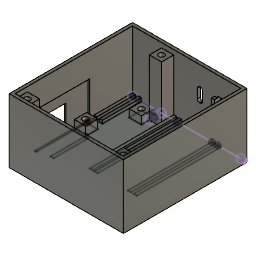
Final_Enclosure (Autodesk Fusion 360 design; units mm, degrees)
Autodesk Fusion 360 part; units mm, degrees
sketch "Sketch1" plane through (0, 0, 0) normal (0, 0, 1) x (1, 0, 0)
  line L0 (0, 0) -> (75, 0)
  line L1 (75, 0) -> (75, 81)
  line L2 (75, 81) -> (0, 81)
  line L3 (0, 81) -> (0, 0)
  dimension "d1" = 81
  dimension "d2" = 75
  constraint horizontal L0
  constraint vertical L1
  constraint horizontal L2
  constraint vertical L3
  constraint coincident L0.start L3.end
  measures "d1" distance of L0.start L2.end
  measures "d2" distance of L0.start L0.end
extrude "Extrude1" add sketch "Sketch1" along normal blind 2 makes body 1
sketch "Sketch2" plane through (0, 0, 2) normal (0, 0, 1) x (-1, 0, 0)
  line L0 (0, -81) -> (0, 0)
  line L1 (0, 0) -> (-75, 0)
  line L2 (-75, 0) -> (-75, -81)
  line L3 (-75, -81) -> (0, -81)
  line L4 (0, 0) -> (-75, 0)
  line L5 (-75, 0) -> (-75, -81)
  line L6 (-75, -81) -> (0, -81)
  line L7 (0, -81) -> (0, 0)
  line L8 (-73, -2) -> (-73, -79)
  line L9 (-73, -79) -> (-2, -79)
  line L10 (-2, -79) -> (-2, -2)
  line L11 (-2, -2) -> (-73, -2)
  dimension "d5" = -2
  constraint horizontal L4
  constraint vertical L5
  constraint horizontal L6
  constraint vertical L7
  constraint coincident L2.end L3.start
  constraint coincident L0.end L1.start
extrude "Extrude2" add sketch "Sketch2" along normal blind 40 bodies 1
sketch "Sketch3" plane through (0, 0, 2) normal (0, 0, 1) x (-1, 0, 0)
  line L0 (-73, -2) -> (-73, -79)
  line L1 (-73, -79) -> (-2, -79)
  line L2 (-2, -79) -> (-2, -2)
  line L3 (-2, -2) -> (-73, -2)
  line L4 (-54, -79) -> (-56, -79)
  line L5 (-56, -79) -> (-56, -24)
  line L6 (-56, -24) -> (-54, -24)
  line L7 (-54, -24) -> (-54, -79)
  line L8 (-57.75, -79) -> (-59.75, -79)
  line L9 (-59.75, -79) -> (-59.75, -24)
  line L10 (-59.75, -24) -> (-57.75, -24)
  line L11 (-57.75, -24) -> (-57.75, -79)
  line L12 (-31, -79) -> (-29, -79)
  line L13 (-29, -79) -> (-29, -24)
  line L14 (-29, -24) -> (-31, -24)
  line L15 (-31, -24) -> (-31, -79)
  line L16 (-34.25, -79) -> (-32.25, -79)
  line L17 (-32.25, -79) -> (-32.25, -24)
  line L18 (-32.25, -24) -> (-34.25, -24)
  line L19 (-34.25, -24) -> (-34.25, -79)
  line L20 (-2, -79) -> (-4, -79)
  line L21 (-4, -79) -> (-4, -53.5)
  line L22 (-4, -53.5) -> (-2, -53.5)
  line L23 (-2, -53.5) -> (-2, -79)
  line L24 (-5.68, -79) -> (-7.68, -79)
  line L25 (-7.68, -79) -> (-7.68, -53.5)
  line L26 (-7.68, -53.5) -> (-5.68, -53.5)
  line L27 (-5.68, -53.5) -> (-5.68, -79)
  line L28 (-9.3, -40.8) -> (-11.3, -40.8)
  line L29 (-11.3, -40.8) -> (-11.3, -18)
  line L30 (-11.3, -18) -> (-9.3, -18)
  line L31 (-9.3, -18) -> (-9.3, -40.8)
  line L32 (-9.3, -40.8) -> (-2, -40.8)
  line L33 (-2, -40.8) -> (-2, -48.8)
  line L34 (-2, -48.8) -> (-9.3, -48.8)
  line L35 (-9.3, -48.8) -> (-9.3, -40.8)
  line L36 (-1, -50.8) -> (-1, -16)
  line L37 (-1, -16) -> (-2, -16)
  line L38 (-2, -16) -> (-2, -48.8)
  line L39 (-1, -50.8) -> (-2, -50.8)
  line L40 (-2, -50.8) -> (-2, -48.8)
  dimension "d8" = 17
  dimension "d9" = 15.25
  dimension "d10" = 2
  dimension "d11" = 2
  dimension "d12" = 55
  dimension "d13" = 25
  dimension "d14" = 23.75
  dimension "d15" = 2
  dimension "d16" = 2
  dimension "d17" = 2
  dimension "d18" = 1.68
  dimension "d19" = 2
  dimension "d20" = 25.5
  dimension "d44" = 7.3
  dimension "d45" = 2
  dimension "d46" = 22.8
  dimension "d47" = 16
  dimension "d48" = 8
  dimension "d49" = 1
  dimension "d50" = 34.8
  dimension "d69" = 2
  constraint horizontal L4
  constraint vertical L5
  constraint horizontal L6
  constraint vertical L7
  constraint coincident L1 L4.start
  constraint horizontal L8
  constraint vertical L9
  constraint horizontal L10
  constraint vertical L11
  constraint coincident L1 L8.start
  constraint horizontal L5.end L10.end
  constraint horizontal L12
  constraint vertical L13
  constraint horizontal L14
  constraint vertical L15
  constraint coincident L1 L12.start
  constraint horizontal L16
  constraint vertical L17
  constraint horizontal L18
  constraint vertical L19
  constraint horizontal L14.end L18.end
  constraint horizontal L6.end L18.end
  constraint horizontal L20
  constraint vertical L21
  constraint horizontal L22
  constraint vertical L23
  constraint coincident L1.end L2.start
  constraint horizontal L24
  constraint vertical L25
  constraint horizontal L26
  constraint vertical L27
  constraint coincident L1 L24.start
  constraint horizontal L21.end L26.end
  constraint horizontal L12.start L16.end
  constraint horizontal L28
  constraint vertical L29
  constraint horizontal L30
  constraint vertical L31
  constraint horizontal L32
  constraint vertical L33
  constraint horizontal L34
  constraint vertical L35
  constraint coincident L2 L33.end
  constraint vertical L36
  constraint horizontal L37
  constraint vertical L38
  constraint coincident L2 L39.end
  constraint perpendicular L2 L39
  measures "d8" distance of L0 L5
  measures "d9" distance of L0 L11
  measures "d10" distance of L5 L7
  measures "d11" distance of L9 L11
  measures "d12" distance of L1 L6
  measures "d13" distance of L5 L15
  measures "d14" distance of L5 L17
  measures "d15" distance of L13 L15
  measures "d16" distance of L17 L19
  measures "d17" distance of L21 L23
  measures "d18" distance of L21 L27
  measures "d19" distance of L25 L27
  measures "d20" distance of L24 L26
  measures "d44" distance of L2 L31
  measures "d45" distance of L29 L31
  measures "d46" distance of L28 L30
  measures "d47" distance of L3 L30
  measures "d48" distance of L28.start L34.end
  measures "d49" distance of L36 L38
  measures "d50" distance of L36.start L36.end
  measures "d69" distance of L30 L37
extrude "Extrude3" add sketch "Sketch3" along normal blind 2 contours L1 L8 L9 L10 L11 | L1 L4 L5 L6 L7 | L1 L2 L20 L21 L22 L23 | L1 L24 L25 L26 L27 bodies 1
extrude "Extrude5" add sketch "Sketch3" along normal blind 3 contours L1 L16 L17 L18 L19 | L1 L12 L13 L14 L15 bodies 1
sketch "Sketch4" plane through (0, 79, 0) normal (0, -1, 0) x (1, 0, 0)
  line L0 (59.75, 4) -> (59.75, 2)
  line L1 (59.75, 2) -> (73, 2)
  line L2 (73, 2) -> (73, 42)
  line L3 (73, 42) -> (2, 42)
  line L4 (2, 42) -> (2, 4)
  line L5 (2, 4) -> (4, 4)
  line L6 (4, 4) -> (4, 2)
  line L7 (4, 2) -> (5.68, 2)
  line L8 (5.68, 2) -> (5.68, 4)
  line L9 (5.68, 4) -> (7.68, 4)
  line L10 (7.68, 4) -> (7.68, 2)
  line L11 (34.25, 2) -> (54, 2)
  line L12 (54, 2) -> (54, 4)
  line L13 (54, 4) -> (56, 4)
  line L14 (56, 4) -> (56, 2)
  line L15 (56, 2) -> (57.75, 2)
  line L16 (57.75, 2) -> (57.75, 4)
  line L17 (57.75, 4) -> (59.75, 4)
  line L18 (57.7, 29.88) -> (68.75, 29.88)
  line L19 (68.75, 29.88) -> (68.75, 20.88)
  line L20 (68.75, 20.88) -> (57.7, 20.88)
  line L21 (57.7, 20.88) -> (57.7, 29.88)
  line L22 (5.68, 7.75) -> (7.61, 7.75)
  line L23 (7.61, 7.75) -> (7.61, 22.05)
  line L24 (7.61, 22.05) -> (5.68, 22.05)
  line L25 (5.68, 22.05) -> (5.68, 7.75)
  line L26 (46, 29.45) -> (46.35, 29.45)
  line L27 (47.85, 27.95) -> (47.85, 21.75)
  line L28 (46.35, 20.25) -> (46, 20.25)
  line L29 (44.5, 21.75) -> (44.5, 27.95)
  line L30 (34.25, 5) -> (34.25, 2)
  line L31 (7.68, 2) -> (29, 2)
  line L32 (29, 2) -> (29, 5)
  line L33 (29, 5) -> (31, 5)
  line L34 (31, 5) -> (31, 2)
  line L35 (31, 2) -> (32.25, 2)
  line L36 (32.25, 2) -> (32.25, 5)
  line L37 (32.25, 5) -> (34.25, 5)
  line L38 (32.25, 2) -> (34.25, 2)
  arc A0 (46, 29.45) -> (44.5, 27.95) centre (46, 27.95) ccw
  arc A1 (47.85, 27.95) -> (46.35, 29.45) centre (46.35, 27.95) ccw
  arc A2 (46.35, 20.25) -> (47.85, 21.75) centre (46.35, 21.75) ccw
  arc A3 (44.5, 21.75) -> (46, 20.25) centre (46, 21.75) ccw
  point P0 (44.5, 29.45)
  point P1 (47.85, 29.45)
  point P2 (44.5, 20.25)
  point P3 (59.75, 2)
  dimension "d23" = 11.05
  dimension "d24" = 9
  dimension "d25" = 18.88
  dimension "d26" = 14.3
  dimension "d27" = 1.93
  dimension "d28" = 5.75
  dimension "d33" = 2.05
  dimension "d39" = 9.2
  dimension "d40" = 3.35
  dimension "d41" = 27.45
  dimension "d42" = 13.5
  dimension "d43" = 1.5
  constraint horizontal L18
  constraint vertical L19
  constraint horizontal L20
  constraint vertical L21
  constraint horizontal L22
  constraint vertical L23
  constraint horizontal L24
  constraint vertical L25
  constraint vertical L8.end L22.start
  constraint horizontal L26
  constraint vertical L27
  constraint horizontal L28
  constraint vertical L29
  constraint coincident P0 L26
  constraint coincident P0 L29
  constraint tangent L26 A0
  constraint tangent L29 A0
  constraint coincident P1 L26
  constraint coincident P1 L27
  constraint tangent L26 A1
  constraint tangent L27 A1
  constraint equal A0 A1
  constraint tangent L27 A2
  constraint tangent L28 A2
  constraint equal A0 A2
  constraint coincident P2 L28
  constraint coincident P2 L29
  constraint tangent L28 A3
  constraint tangent L29 A3
  constraint equal A0 A3
  measures "d23" distance of L18.start L18.end
  measures "d24" distance of L18.start L20.end
  measures "d25" distance of L15 L20
  measures "d26" distance of L22.end L23.end
  measures "d27" distance of L23.end L24.end
  measures "d28" distance of L7 L22
  measures "d33" distance of L21 P3
  measures "d39" distance of P0 P2
  measures "d40" distance of P0 P1
  measures "d41" distance of L26 L38
  measures "d42" distance of L29 L34
  measures "d43" radius of A0
extrude "Extrude4" cut sketch "Sketch4" against normal blind 5 contours L18 L19 L20 L21 | L26 L27 L28 L29 A0 A1 A2 A3 bodies 1
sketch "Sketch5" plane through (0, 79, 0) normal (0, -1, 0) x (1, 0, 0)
  line L0 (47.85, 27.95) -> (47.85, 21.75)
  line L1 (46.35, 20.25) -> (46, 20.25)
  line L2 (44.5, 21.75) -> (44.5, 27.95)
  line L3 (46, 29.45) -> (46.35, 29.45)
  line L4 (68.75, 29.88) -> (68.75, 20.88)
  line L5 (68.75, 20.88) -> (57.7, 20.88)
  line L6 (57.7, 20.88) -> (57.7, 29.88)
  line L7 (57.7, 29.88) -> (68.75, 29.88)
  line L8 (34.25, 5) -> (34.25, 2)
  line L9 (34.25, 2) -> (54, 2)
  line L10 (54, 2) -> (54, 4)
  line L11 (54, 4) -> (56, 4)
  line L12 (56, 4) -> (56, 2)
  line L13 (56, 2) -> (57.75, 2)
  line L14 (57.75, 2) -> (57.75, 4)
  line L15 (57.75, 4) -> (59.75, 4)
  line L16 (59.75, 4) -> (59.75, 2)
  line L17 (59.75, 2) -> (73, 2)
  line L18 (73, 2) -> (73, 42)
  line L19 (73, 42) -> (2, 42)
  line L20 (2, 42) -> (2, 4)
  line L21 (2, 4) -> (4, 4)
  line L22 (4, 4) -> (4, 2)
  line L23 (4, 2) -> (5.68, 2)
  line L24 (5.68, 2) -> (5.68, 4)
  line L25 (5.68, 4) -> (7.68, 4)
  line L26 (7.68, 4) -> (7.68, 2)
  line L27 (7.68, 2) -> (29, 2)
  line L28 (29, 2) -> (29, 5)
  line L29 (29, 5) -> (31, 5)
  line L30 (31, 5) -> (31, 2)
  line L31 (31, 2) -> (32.25, 2)
  line L32 (32.25, 2) -> (32.25, 5)
  line L33 (32.25, 5) -> (34.25, 5)
  line L34 (57.7, 21.88) -> (55.7, 21.88)
  line L35 (55.7, 21.88) -> (55.7, 28.88)
  line L36 (55.7, 28.88) -> (57.7, 28.88)
  line L37 (57.7, 28.88) -> (57.7, 21.88)
  arc A0 (46, 29.45) -> (44.5, 27.95) centre (46, 27.95) ccw
  arc A1 (47.85, 27.95) -> (46.35, 29.45) centre (46.35, 27.95) ccw
  arc A2 (46.35, 20.25) -> (47.85, 21.75) centre (46.35, 21.75) ccw
  arc A3 (44.5, 21.75) -> (46, 20.25) centre (46, 21.75) ccw
  dimension "d34" = 1
  dimension "d35" = 1
  dimension "d36" = 2
  constraint horizontal L34
  constraint vertical L35
  constraint horizontal L36
  constraint vertical L37
  constraint coincident L6 L34.start
  measures "d34" distance of L7 L36
  measures "d35" distance of L5 L34
  measures "d36" distance of L35.end L36.end
extrude "Extrude6" add sketch "Sketch5" along normal blind 2 contours L6 L34 L35 L36 L37 bodies 1
extrude "Extrude7" add sketch "Sketch3" along normal blind 2 contours L28 L29 L30 L31 bodies 1
extrude "Extrude8" add sketch "Sketch3" along normal blind 5.9 contours L2 L32 L33 L34 L35 L38 bodies 1
extrude "Extrude9" cut sketch "Sketch3" along normal blind 24 contours L2 L33 L36 L37 L38 L39 L40 bodies 1
sketch "Sketch7" plane through (1, 0, 0) normal (1, 0, 0) x (0, 1, 0)
  line L0 (16, 2) -> (50.8, 2)
  line L1 (50.8, 26) -> (16, 26)
  line L2 (16, 26) -> (16, 2)
  line L3 (16, 26) -> (50.8, 26)
  line L4 (50.8, 26) -> (50.8, 2)
  line L5 (50.8, 2) -> (16, 2)
  line L6 (16, 2) -> (16, 26)
  line L7 (23.5, 19) -> (36.3, 19)
  line L8 (36.3, 19) -> (36.3, 6)
  line L9 (36.3, 6) -> (23.5, 6)
  line L10 (23.5, 6) -> (23.5, 19)
  line L11 (79, 2) -> (24, 2)
  line L12 (50.8, 2) -> (50.8, 26)
  dimension "d58" = 7
  dimension "d59" = 4
  dimension "d60" = 7.5
  dimension "d61" = 14.5
  constraint horizontal L3
  constraint vertical L4
  constraint horizontal L5
  constraint vertical L6
  constraint coincident L0.end L4.end
  constraint coincident L1.end L2.start
  constraint horizontal L7
  constraint vertical L8
  constraint horizontal L9
  constraint vertical L10
  measures "d58" distance of L3 L7
  measures "d59" distance of L9 L11
  measures "d60" distance of L6 L10
  measures "d61" distance of L4 L8
extrude "Extrude10" cut sketch "Sketch7" against normal blind 5 contours L7 L8 L9 L10 bodies 1
sketch "Sketch8" plane through (0, 0, 7.9) normal (0, 0, 1) x (-1, 0, 0)
  line L0 (-9.3, -40.8) -> (-9.3, -48.8)
  line L1 (-9.3, -48.8) -> (-2, -48.8)
  line L2 (-2, -48.8) -> (-2, -40.8)
  line L3 (-2, -40.8) -> (-9.3, -40.8)
  circle A0 centre (-5.2, -44.8) radius 1.825
  line L4 (-2, -48.8) -> (-9.3, -48.8)
  line L5 (-9.3, -48.8) -> (-9.3, -40.8)
  dimension "d64" = 3.65
  dimension "d65" = 4
  dimension "d66" = 4.1
  measures "d64" diameter of A0
  measures "d65" distance of A0.centre L4
  measures "d66" distance of A0.centre L5
extrude "Extrude11" cut sketch "Sketch8" against normal blind 6 contours A0 bodies 1
sketch "Sketch9" plane through (0, 0, 2) normal (0, 0, 1) x (-1, 0, 0)
  line L0 (-2, -2) -> (-10, -2)
  line L1 (-10, -2) -> (-10, -10)
  line L2 (-10, -10) -> (-2, -10)
  line L3 (-2, -10) -> (-2, -2)
  line L4 (-73, -2) -> (-65, -2)
  line L5 (-65, -2) -> (-65, -10)
  line L6 (-65, -10) -> (-73, -10)
  line L7 (-73, -10) -> (-73, -2)
  line L8 (-29, -79) -> (-21, -79)
  line L9 (-21, -79) -> (-21, -71)
  line L10 (-21, -71) -> (-29, -71)
  line L11 (-29, -71) -> (-29, -79)
  line L12 (-29, -79) -> (-29, -24)
  line L13 (-2, -79) -> (-2, -2)
  line L14 (-2, -2) -> (-73, -2)
  line L15 (-29, -24) -> (-31, -24)
  line L16 (-73, -79) -> (-2, -79)
  line L17 (-59.75, -24) -> (-57.75, -24)
  line L18 (-73, -2) -> (-73, -79)
  point P0 (-11.3, -18)
  dimension "d70" = 8
  dimension "d71" = 8
  dimension "d73" = 8
  dimension "d74" = 8
  dimension "d77" = 8
  dimension "d78" = 8
  constraint horizontal L0
  constraint vertical L1
  constraint horizontal L2
  constraint vertical L3
  constraint horizontal L4
  constraint vertical L5
  constraint horizontal L6
  constraint vertical L7
  constraint horizontal L8
  constraint vertical L9
  constraint horizontal L10
  constraint vertical L11
  constraint collinear L3 L13
  constraint collinear L0 L14
  constraint collinear L8 L16
  constraint collinear L4 L14
  constraint collinear L7 L18
  constraint collinear L11 L12
  measures "d70" distance of L9.end L10.end
  measures "d71" distance of L8.end L9.end
  measures "d73" distance of L0.end L1.end
  measures "d74" distance of L1.end L2.end
  measures "d77" distance of L4.end L5.end
  measures "d78" distance of L5.end L6.end
extrude "Extrude12" add sketch "Sketch9" along normal blind 37 separate body contours L0 L1 L2 L3 L13 L14 | L4 L5 L6 L7 L14 L18 | L8 L9 L10 L11 L12 L16 makes body 2 at (67.6667, 10, 14.3333) makes body 3 at (2, 7.3333, 14.3333) makes body 4 at (29, 73.6667, 14.3333)
sketch "Sketch10" plane through (0, 0, 39) normal (0, 0, 1) x (-1, 0, 0)
  line L0 (-65, -2) -> (-73, -2)
  line L1 (-73, -2) -> (-73, -10)
  line L2 (-73, -10) -> (-65, -10)
  line L3 (-65, -10) -> (-65, -2)
  circle A0 centre (-69, -6) radius 1.825
  circle A1 centre (-6, -6) radius 1.825
  circle A2 centre (-25, -75) radius 1.825
  line L4 (-29, -71) -> (-29, -79)
  line L5 (-21, -71) -> (-29, -71)
  line L6 (-10, -2) -> (-10, -10)
  line L7 (-10, -10) -> (-2, -10)
  dimension "d82" = 4
  dimension "d83" = 4
  dimension "d84" = 3.65
  dimension "d85" = 3.65
  dimension "d86" = 4
  dimension "d87" = 4
  dimension "d88" = 3.65
  dimension "d89" = 4
  dimension "d90" = 4
  measures "d82" distance of A2.centre L4
  measures "d83" distance of A2.centre L5
  measures "d84" diameter of A2
  measures "d85" diameter of A0
  measures "d86" distance of L3 A0.centre
  measures "d87" distance of L2 A0.centre
  measures "d88" diameter of A1
  measures "d89" distance of A1.centre L6
  measures "d90" distance of A1.centre L7
extrude "Extrude13" cut sketch "Sketch10" against normal blind 6 contours A0 | A1 | A2 bodies 2 3 4
sketch "Sketch13" plane through (0, 0, 2) normal (0, 0, 1) x (-1, 0, 0)
  line L0 (-21, -79) -> (-16.5, -79)
  line L1 (-16.5, -79) -> (-16.5, -75.85)
  line L2 (-16.5, -75.85) -> (-21, -75.85)
  line L3 (-21, -75.85) -> (-21, -79)
  line L4 (-21, -79) -> (-21, -71)
  line L5 (-73, -79) -> (-2, -79)
  line L6 (-21, -73.8) -> (-13, -73.8)
  line L7 (-13, -73.8) -> (-13, -65.8)
  line L8 (-13, -65.8) -> (-21, -65.8)
  line L9 (-21, -65.8) -> (-21, -73.8)
  dimension "d101" = 4.5
  dimension "d102" = 3.15
  dimension "d104" = 8
  dimension "d105" = 8
  dimension "d106" = 2.05
  constraint horizontal L0
  constraint vertical L1
  constraint horizontal L2
  constraint vertical L3
  constraint collinear L3 L4
  constraint collinear L0 L5
  constraint horizontal L6
  constraint vertical L7
  constraint horizontal L8
  constraint vertical L9
  constraint coincident L4 L6.start
  measures "d101" distance of L1.end L2.end
  measures "d102" distance of L0.end L1.end
  measures "d104" distance of L6.start L6.end
  measures "d105" distance of L6.end L7.end
  measures "d106" distance of L2 L6
extrude "Extrude15" add sketch "Sketch13" along normal blind 5 contours L4 L6 L7 L8 L9 bodies 1 2 3 4
extrude "Extrude16" add sketch "Sketch13" along normal blind 2.5 contours L0 L1 L2 L3 L4 L5 bodies 1 2 3
sketch "Sketch14" plane through (0, 79, 0) normal (0, -1, 0) x (1, 0, 0)
  line L0 (44.5, 21.75) -> (44.5, 27.95)
  arc A0 (46, 29.45) -> (44.5, 27.95) centre (46, 27.95) ccw
  line L1 (46, 29.45) -> (46.35, 29.45)
  arc A1 (47.85, 27.95) -> (46.35, 29.45) centre (46.35, 27.95) ccw
  line L2 (47.85, 27.95) -> (47.85, 21.75)
  arc A2 (46.35, 20.25) -> (47.85, 21.75) centre (46.35, 21.75) ccw
  line L3 (46.35, 20.25) -> (46, 20.25)
  arc A3 (44.5, 21.75) -> (46, 20.25) centre (46, 21.75) ccw
  line L4 (57.7, 21.88) -> (55.7, 21.88)
  line L5 (55.7, 21.88) -> (55.7, 28.88)
  line L6 (55.7, 28.88) -> (57.7, 28.88)
  line L7 (57.7, 28.88) -> (57.7, 29.88)
  line L8 (57.7, 29.88) -> (68.75, 29.88)
  line L9 (68.75, 29.88) -> (68.75, 20.88)
  line L10 (68.75, 20.88) -> (57.7, 20.88)
  line L11 (57.7, 20.88) -> (57.7, 21.88)
  line L12 (16.5, 2) -> (16.5, 4.5)
  line L13 (16.5, 4.5) -> (21, 4.5)
  line L14 (21, 4.5) -> (21, 39)
  line L15 (21, 39) -> (29, 39)
  line L16 (29, 39) -> (29, 5)
  line L17 (29, 5) -> (31, 5)
  line L18 (31, 5) -> (31, 2)
  line L19 (31, 2) -> (32.25, 2)
  line L20 (32.25, 2) -> (32.25, 5)
  line L21 (32.25, 5) -> (34.25, 5)
  line L22 (34.25, 5) -> (34.25, 2)
  line L23 (34.25, 2) -> (54, 2)
  line L24 (54, 2) -> (54, 4)
  line L25 (54, 4) -> (56, 4)
  line L26 (56, 4) -> (56, 2)
  line L27 (56, 2) -> (57.75, 2)
  line L28 (57.75, 2) -> (57.75, 4)
  line L29 (57.75, 4) -> (59.75, 4)
  line L30 (59.75, 4) -> (59.75, 2)
  line L31 (59.75, 2) -> (73, 2)
  line L32 (73, 2) -> (73, 42)
  line L33 (73, 42) -> (2, 42)
  line L34 (2, 42) -> (2, 4)
  line L35 (2, 4) -> (4, 4)
  line L36 (4, 4) -> (4, 2)
  line L37 (4, 2) -> (5.68, 2)
  line L38 (5.68, 2) -> (5.68, 4)
  line L39 (5.68, 4) -> (7.68, 4)
  line L40 (7.68, 4) -> (7.68, 2)
  line L41 (7.68, 2) -> (16.5, 2)
  circle A4 centre (18.75, 6.75) radius 1.25
  line L42 (13, 2) -> (21, 2)
  dimension "d111" = 2.25
  dimension "d112" = 4.75
  dimension "d113" = 2.5
  measures "d111" distance of L14 A4.centre
  measures "d112" distance of A4.centre L42
  measures "d113" diameter of A4
extrude "Extrude17" cut sketch "Sketch14" against normal blind 3 contours A4 bodies 1
sketch "Sketch16" plane through (0, 0, 7) normal (0, 0, 1) x (-1, 0, 0)
  line L0 (-21, -65.8) -> (-21, -71)
  line L1 (-21, -71) -> (-21, -73.8)
  line L2 (-21, -73.8) -> (-13, -73.8)
  line L3 (-13, -73.8) -> (-13, -65.8)
  line L4 (-13, -65.8) -> (-21, -65.8)
  circle A0 centre (-17, -69.8) radius 1.825
  line L5 (-13, -65.8) -> (-21, -65.8)
  line L6 (-21, -65.8) -> (-21, -73.8)
  dimension "d116" = 4
  dimension "d117" = 4
  dimension "d118" = 3.65
  measures "d116" distance of A0.centre L5
  measures "d117" distance of A0.centre L6
  measures "d118" diameter of A0
extrude "Extrude18" cut sketch "Sketch16" against normal blind 4.5 contours A0 bodies 1
